Autodesk Inventor part; units mm, degrees
(part 2 of 3)
  line L1044 (421.44, -35) -> (424.615, -35) projected
  line L1045 (421.44, -45) -> (421.44, -35) projected
  line L1046 (424.615, -45) -> (421.44, -45) projected
  line L1047 (424.615, -45) -> (424.615, -55) projected
  line L1048 (421.44, -55) -> (424.615, -55) projected
  line L1049 (421.44, -65) -> (421.44, -55) projected
  line L1050 (424.615, -65) -> (421.44, -65) projected
  line L1051 (424.615, -65) -> (424.615, -75) projected
  line L1052 (421.44, -75) -> (424.615, -75) projected
  line L1053 (421.44, -75) -> (421.44, -86.825) projected
  line L1054 (421.44, -86.825) -> (426.44, -86.825) projected
  line L1055 (426.44, -86.825) -> (426.44, -90) projected
  line L1056 (426.44, -90) -> (436.44, -90) projected
  line L1057 (436.44, -90) -> (436.44, -86.825) projected
  line L1058 (436.44, -86.825) -> (446.44, -86.825) projected
  line L1059 (446.44, -86.825) -> (446.44, -90) projected
  line L1060 (446.44, -90) -> (456.44, -90) projected
  line L1061 (456.44, -90) -> (456.44, -86.825) projected
  line L1062 (456.44, -86.825) -> (466.44, -86.825) projected
  line L1063 (466.44, -86.825) -> (466.44, -90) projected
  line L1064 (466.44, -90) -> (476.44, -90) projected
  line L1065 (476.44, -90) -> (476.44, -86.825) projected
  line L1066 (476.44, -86.825) -> (486.44, -86.825) projected
  line L1067 (486.44, -86.825) -> (486.44, -90) projected
  line L1068 (486.44, -90) -> (496.44, -90) projected
  line L1069 (496.44, -90) -> (496.44, -86.825) projected
  line L1070 (496.44, -86.825) -> (506.44, -86.825) projected
  line L1071 (506.44, -86.825) -> (506.44, -90) projected
  line L1072 (506.44, -90) -> (516.44, -90) projected
  line L1073 (516.44, -90) -> (516.44, -86.825) projected
  line L1074 (516.44, -86.825) -> (526.44, -86.825) projected
  line L1075 (526.44, -86.825) -> (526.44, -90) projected
  line L1076 (526.44, -90) -> (536.44, -90) projected
  line L1077 (536.44, -90) -> (536.44, -86.825) projected
  line L1078 (536.44, -86.825) -> (541.44, -86.825) projected
  line L1079 (541.44, -86.825) -> (541.44, -75) projected
  line L1080 (541.44, -75) -> (538.265, -75) projected
  line L1081 (538.265, -75) -> (538.265, -65) projected
  line L1082 (538.265, -65) -> (541.44, -65) projected
  line L1083 (541.44, -65) -> (541.44, -55) projected
  line L1084 (541.44, -55) -> (538.265, -55) projected
  line L1085 (538.265, -55) -> (538.265, -51.5) projected
  line L1086 (538.265, -51.5) -> (536.265, -51.5) projected
  line L1087 (536.265, -51.5) -> (536.265, -52.75) projected
  line L1088 (536.265, -52.75) -> (533.765, -52.75) projected
  line L1089 (533.765, -52.75) -> (533.765, -51.5) projected
  line L1090 (533.765, -51.5) -> (527.44, -51.5) projected
  line L1091 (527.44, -51.5) -> (527.44, -48.5) projected
  line L1092 (527.44, -48.5) -> (533.765, -48.5) projected
  line L1093 (533.765, -48.5) -> (533.765, -47.25) projected
  line L1094 (533.765, -47.25) -> (536.265, -47.25) projected
  line L1095 (536.265, -47.25) -> (536.265, -48.5) projected
  circle A30 centre (504.4372, -27.4451) radius 3 projected
  circle A31 centre (458.4428, 54) radius 3 projected
  circle A32 centre (504.4372, 27.4451) radius 3 projected
  circle A33 centre (458.4428, -54) radius 3 projected
  circle A34 centre (466.44, 8.175) radius 11 projected
  line L1096 (541.56, 86.945) -> (541.56, 74.88)
  line L1097 (541.56, 74.88) -> (538.385, 74.88)
  line L1098 (538.385, 74.88) -> (538.385, 65.12)
  line L1099 (538.385, 65.12) -> (541.56, 65.12)
  line L1100 (541.56, 65.12) -> (541.56, 54.88)
  line L1101 (541.56, 54.88) -> (538.385, 54.88)
  line L1102 (538.385, 54.88) -> (538.385, 51.38)
  line L1103 (538.385, 51.38) -> (536.145, 51.38)
  line L1104 (536.145, 51.38) -> (536.145, 52.63)
  line L1105 (536.145, 52.63) -> (533.885, 52.63)
  line L1106 (533.885, 52.63) -> (533.885, 51.38)
  line L1107 (533.885, 51.38) -> (527.56, 51.38)
  line L1108 (527.56, 51.38) -> (527.56, 48.62)
  line L1109 (527.56, 48.62) -> (533.885, 48.62)
  line L1110 (533.885, 48.62) -> (533.885, 47.37)
  line L1111 (533.885, 47.37) -> (536.145, 47.37)
  line L1112 (536.145, 47.37) -> (536.145, 48.62)
  line L1113 (536.145, 48.62) -> (538.385, 48.62)
  line L1114 (538.385, 48.62) -> (538.385, 45.12)
  line L1115 (538.385, 45.12) -> (541.56, 45.12)
  line L1116 (541.56, 45.12) -> (541.56, 34.88)
  line L1117 (541.56, 34.88) -> (538.385, 34.88)
  line L1118 (538.385, 34.88) -> (538.385, 25.12)
  line L1119 (538.385, 25.12) -> (541.56, 25.12)
  line L1120 (541.56, 25.12) -> (541.56, 14.88)
  line L1121 (541.56, 14.88) -> (538.385, 14.88)
  line L1122 (538.385, 14.88) -> (538.385, 5.12)
  line L1123 (538.385, 5.12) -> (541.56, 5.12)
  line L1124 (541.56, 5.12) -> (541.56, -5.12)
  line L1125 (541.56, -5.12) -> (538.385, -5.12)
  line L1126 (538.385, -5.12) -> (538.385, -14.88)
  line L1127 (538.385, -14.88) -> (541.56, -14.88)
  line L1128 (541.56, -14.88) -> (541.56, -25.12)
  line L1129 (541.56, -25.12) -> (538.385, -25.12)
  line L1130 (538.385, -25.12) -> (538.385, -34.88)
  line L1131 (538.385, -34.88) -> (541.56, -34.88)
  line L1132 (541.56, -34.88) -> (541.56, -45.12)
  line L1133 (541.56, -45.12) -> (538.385, -45.12)
  line L1134 (538.385, -45.12) -> (538.385, -48.62)
  line L1135 (538.385, -48.62) -> (536.145, -48.62)
  line L1136 (536.145, -48.62) -> (536.145, -47.37)
  line L1137 (536.145, -47.37) -> (533.885, -47.37)
  line L1138 (533.885, -47.37) -> (533.885, -48.62)
  line L1139 (533.885, -48.62) -> (527.56, -48.62)
  line L1140 (527.56, -48.62) -> (527.56, -51.38)
  line L1141 (527.56, -51.38) -> (533.885, -51.38)
  line L1142 (533.885, -51.38) -> (533.885, -52.63)
  line L1143 (533.885, -52.63) -> (536.145, -52.63)
  line L1144 (536.145, -52.63) -> (536.145, -51.38)
  line L1145 (536.145, -51.38) -> (538.385, -51.38)
  line L1146 (538.385, -51.38) -> (538.385, -54.88)
  line L1147 (538.385, -54.88) -> (541.56, -54.88)
  line L1148 (541.56, -54.88) -> (541.56, -65.12)
  line L1149 (541.56, -65.12) -> (538.385, -65.12)
  line L1150 (538.385, -65.12) -> (538.385, -74.88)
  line L1151 (538.385, -74.88) -> (541.56, -74.88)
  line L1152 (541.56, -74.88) -> (541.56, -86.945)
  line L1153 (541.56, -86.945) -> (536.56, -86.945)
  line L1154 (536.56, -86.945) -> (536.56, -90.12)
  line L1155 (536.56, -90.12) -> (526.32, -90.12)
  line L1156 (526.32, -90.12) -> (526.32, -86.945)
  line L1157 (526.32, -86.945) -> (516.56, -86.945)
  line L1158 (516.56, -86.945) -> (516.56, -90.12)
  line L1159 (516.56, -90.12) -> (506.32, -90.12)
  line L1160 (506.32, -90.12) -> (506.32, -86.945)
  line L1161 (506.32, -86.945) -> (496.56, -86.945)
  line L1162 (496.56, -86.945) -> (496.56, -90.12)
  line L1163 (496.56, -90.12) -> (486.32, -90.12)
  line L1164 (486.32, -90.12) -> (486.32, -86.945)
  line L1165 (486.32, -86.945) -> (476.56, -86.945)
  line L1166 (476.56, -86.945) -> (476.56, -90.12)
  line L1167 (476.56, -90.12) -> (466.32, -90.12)
  line L1168 (466.32, -90.12) -> (466.32, -86.945)
  line L1169 (466.32, -86.945) -> (456.56, -86.945)
  line L1170 (456.56, -86.945) -> (456.56, -90.12)
  line L1171 (456.56, -90.12) -> (446.32, -90.12)
  line L1172 (446.32, -90.12) -> (446.32, -86.945)
  line L1173 (446.32, -86.945) -> (436.56, -86.945)
  line L1174 (436.56, -86.945) -> (436.56, -90.12)
  line L1175 (436.56, -90.12) -> (426.32, -90.12)
  line L1176 (426.32, -90.12) -> (426.32, -86.945)
  line L1177 (426.32, -86.945) -> (421.32, -86.945)
  line L1178 (421.32, -86.945) -> (421.32, -74.88)
  line L1179 (421.32, -74.88) -> (424.495, -74.88)
  line L1180 (424.495, -74.88) -> (424.495, -65.12)
  line L1181 (424.495, -65.12) -> (421.32, -65.12)
  line L1182 (421.32, -65.12) -> (421.32, -54.88)
  line L1183 (421.32, -54.88) -> (424.495, -54.88)
  line L1184 (424.495, -54.88) -> (424.495, -45.12)
  line L1185 (424.495, -45.12) -> (421.32, -45.12)
  line L1186 (421.32, -45.12) -> (421.32, -34.88)
  line L1187 (421.32, -34.88) -> (424.495, -34.88)
  line L1188 (424.495, -34.88) -> (424.495, -25.12)
  line L1189 (424.495, -25.12) -> (421.32, -25.12)
  line L1190 (421.32, -25.12) -> (421.32, -14.88)
  line L1191 (421.32, -14.88) -> (424.495, -14.88)
  line L1192 (424.495, -14.88) -> (424.495, -5.12)
  line L1193 (424.495, -5.12) -> (421.32, -5.12)
  line L1194 (421.32, -5.12) -> (421.32, 5.12)
  line L1195 (421.32, 5.12) -> (424.495, 5.12)
  line L1196 (424.495, 5.12) -> (424.495, 14.88)
  line L1197 (424.495, 14.88) -> (421.32, 14.88)
  line L1198 (421.32, 14.88) -> (421.32, 25.12)
  line L1199 (421.32, 25.12) -> (424.495, 25.12)
  line L1200 (424.495, 25.12) -> (424.495, 34.88)
  line L1201 (424.495, 34.88) -> (421.32, 34.88)
  line L1202 (421.32, 34.88) -> (421.32, 45.12)
  line L1203 (421.32, 45.12) -> (424.495, 45.12)
  line L1204 (424.495, 45.12) -> (424.495, 54.88)
  line L1205 (424.495, 54.88) -> (421.32, 54.88)
  line L1206 (421.32, 54.88) -> (421.32, 65.12)
  line L1207 (421.32, 65.12) -> (424.495, 65.12)
  line L1208 (424.495, 65.12) -> (424.495, 74.88)
  line L1209 (424.495, 74.88) -> (421.32, 74.88)
  line L1210 (421.32, 74.88) -> (421.32, 86.945)
  line L1211 (421.32, 86.945) -> (426.32, 86.945)
  line L1212 (426.32, 86.945) -> (426.32, 90.12)
  line L1213 (426.32, 90.12) -> (436.56, 90.12)
  line L1214 (436.56, 90.12) -> (436.56, 86.945)
  line L1215 (436.56, 86.945) -> (446.32, 86.945)
  line L1216 (446.32, 86.945) -> (446.32, 90.12)
  line L1217 (446.32, 90.12) -> (456.56, 90.12)
  line L1218 (456.56, 90.12) -> (456.56, 86.945)
  line L1219 (456.56, 86.945) -> (466.32, 86.945)
  line L1220 (466.32, 86.945) -> (466.32, 90.12)
  line L1221 (466.32, 90.12) -> (476.56, 90.12)
  line L1222 (476.56, 90.12) -> (476.56, 86.945)
  line L1223 (476.56, 86.945) -> (486.32, 86.945)
  line L1224 (486.32, 86.945) -> (486.32, 90.12)
  line L1225 (486.32, 90.12) -> (496.56, 90.12)
  line L1226 (496.56, 90.12) -> (496.56, 86.945)
  line L1227 (496.56, 86.945) -> (506.32, 86.945)
  line L1228 (506.32, 86.945) -> (506.32, 90.12)
  line L1229 (506.32, 90.12) -> (516.56, 90.12)
  line L1230 (516.56, 90.12) -> (516.56, 86.945)
  line L1231 (516.56, 86.945) -> (526.32, 86.945)
  line L1232 (526.32, 86.945) -> (526.32, 90.12)
  line L1233 (526.32, 90.12) -> (536.56, 90.12)
  line L1234 (536.56, 90.12) -> (536.56, 86.945)
  line L1235 (536.56, 86.945) -> (541.56, 86.945)
  circle A35 centre (527.16, 0) radius 0.958
  circle A36 centre (519.54, 0) radius 0.958
  line L1236 (525.135, -13.215) -> (521.565, -13.215)
  line L1237 (521.565, -13.215) -> (521.565, -2.025)
  line L1238 (521.565, -2.025) -> (525.135, -2.025)
  line L1239 (525.135, -2.025) -> (525.135, -13.215)
  circle A37 centre (527.16, -15.24) radius 0.958
  circle A38 centre (519.54, -15.24) radius 1.198
  circle A39 centre (504.4372, 27.4451) radius 2.88
  circle A40 centre (504.4372, -27.4451) radius 2.88
  circle A41 centre (533.716, -59.1479) radius 0.958
  circle A42 centre (498.716, -59.1479) radius 0.958
  circle A43 centre (458.4428, 54) radius 2.88
  circle A44 centre (466.44, 8.175) radius 10.88
  line L1240 (404.895, -13.335) -> (401.085, -13.335) projected
  line L1241 (401.085, -13.335) -> (401.085, -1.905) projected
  line L1242 (401.085, -1.905) -> (404.895, -1.905) projected
  line L1243 (404.895, -1.905) -> (404.895, -13.335) projected
  circle A45 centre (399.18, -15.24) radius 1.078 projected
  circle A46 centre (406.8, 0) radius 1.078 projected
  circle A47 centre (406.8, -15.24) radius 1.078 projected
  circle A48 centre (399.18, 0) radius 1.078 projected
  line L1244 (415.905, -48.5) -> (417.905, -48.5) projected
  line L1245 (417.905, -48.5) -> (417.905, -45) projected
  line L1246 (417.905, -45) -> (421.08, -45) projected
  line L1247 (421.08, -45) -> (421.08, -35) projected
  line L1248 (421.08, -35) -> (417.905, -35) projected
  line L1249 (417.905, -35) -> (417.905, -25) projected
  line L1250 (417.905, -25) -> (421.08, -25) projected
  line L1251 (421.08, -25) -> (421.08, -15) projected
  line L1252 (421.08, -15) -> (417.905, -15) projected
  line L1253 (417.905, -15) -> (417.905, -5) projected
  line L1254 (417.905, -5) -> (421.08, -5) projected
  line L1255 (421.08, -5) -> (421.08, 5) projected
  line L1256 (421.08, 5) -> (417.905, 5) projected
  line L1257 (417.905, 5) -> (417.905, 15) projected
  line L1258 (417.905, 15) -> (421.08, 15) projected
  line L1259 (421.08, 15) -> (421.08, 25) projected
  line L1260 (421.08, 25) -> (417.905, 25) projected
  line L1261 (417.905, 25) -> (417.905, 35) projected
  line L1262 (417.905, 35) -> (421.08, 35) projected
  line L1263 (421.08, 35) -> (421.08, 45) projected
  line L1264 (421.08, 45) -> (417.905, 45) projected
  line L1265 (417.905, 45) -> (417.905, 48.5) projected
  line L1266 (417.905, 48.5) -> (415.905, 48.5) projected
  line L1267 (415.905, 48.5) -> (415.905, 47.25) projected
  line L1268 (415.905, 47.25) -> (413.405, 47.25) projected
  line L1269 (413.405, 47.25) -> (413.405, 48.5) projected
  line L1270 (413.405, 48.5) -> (407.08, 48.5) projected
  line L1271 (407.08, 48.5) -> (407.08, 51.5) projected
  line L1272 (407.08, 51.5) -> (413.405, 51.5) projected
  line L1273 (413.405, 51.5) -> (413.405, 52.75) projected
  line L1274 (413.405, 52.75) -> (415.905, 52.75) projected
  line L1275 (415.905, 52.75) -> (415.905, 51.5) projected
  line L1276 (415.905, 51.5) -> (417.905, 51.5) projected
  line L1277 (417.905, 51.5) -> (417.905, 55) projected
  line L1278 (417.905, 55) -> (421.08, 55) projected
  line L1279 (421.08, 55) -> (421.08, 65) projected
  line L1280 (421.08, 65) -> (417.905, 65) projected
  line L1281 (417.905, 65) -> (417.905, 75) projected
  line L1282 (417.905, 75) -> (421.08, 75) projected
  line L1283 (421.08, 75) -> (421.08, 86.825) projected
  line L1284 (416.08, 86.825) -> (421.08, 86.825) projected
  line L1285 (416.08, 90) -> (416.08, 86.825) projected
  line L1286 (406.08, 90) -> (416.08, 90) projected
  line L1287 (406.08, 86.825) -> (406.08, 90) projected
  line L1288 (406.08, 86.825) -> (396.08, 86.825) projected
  line L1289 (396.08, 90) -> (396.08, 86.825) projected
  line L1290 (386.08, 90) -> (396.08, 90) projected
  line L1291 (386.08, 86.825) -> (386.08, 90) projected
  line L1292 (386.08, 86.825) -> (376.08, 86.825) projected
  line L1293 (376.08, 90) -> (376.08, 86.825) projected
  line L1294 (366.08, 90) -> (376.08, 90) projected
  line L1295 (366.08, 86.825) -> (366.08, 90) projected
  line L1296 (366.08, 86.825) -> (356.08, 86.825) projected
  line L1297 (356.08, 90) -> (356.08, 86.825) projected
  line L1298 (346.08, 90) -> (356.08, 90) projected
  line L1299 (346.08, 86.825) -> (346.08, 90) projected
  line L1300 (346.08, 86.825) -> (336.08, 86.825) projected
  line L1301 (336.08, 90) -> (336.08, 86.825) projected
  line L1302 (326.08, 90) -> (336.08, 90) projected
  line L1303 (326.08, 86.825) -> (326.08, 90) projected
  line L1304 (326.08, 86.825) -> (316.08, 86.825) projected
  line L1305 (316.08, 90) -> (316.08, 86.825) projected
  line L1306 (306.08, 90) -> (316.08, 90) projected
  line L1307 (306.08, 86.825) -> (306.08, 90) projected
  line L1308 (306.08, 86.825) -> (301.08, 86.825) projected
  line L1309 (301.08, 75) -> (301.08, 86.825) projected
  line L1310 (304.255, 75) -> (301.08, 75) projected
  line L1311 (304.255, 75) -> (304.255, 65) projected
  line L1312 (301.08, 65) -> (304.255, 65) projected
  line L1313 (301.08, 55) -> (301.08, 65) projected
  line L1314 (304.255, 55) -> (301.08, 55) projected
  line L1315 (304.255, 55) -> (304.255, 45) projected
  line L1316 (301.08, 45) -> (304.255, 45) projected
  line L1317 (301.08, 35) -> (301.08, 45) projected
  line L1318 (304.255, 35) -> (301.08, 35) projected
  line L1319 (304.255, 35) -> (304.255, 25) projected
  line L1320 (301.08, 25) -> (304.255, 25) projected
  line L1321 (301.08, 15) -> (301.08, 25) projected
  line L1322 (304.255, 15) -> (301.08, 15) projected
  line L1323 (304.255, 15) -> (304.255, 5) projected
  line L1324 (301.08, 5) -> (304.255, 5) projected
  line L1325 (301.08, -5) -> (301.08, 5) projected
  line L1326 (304.255, -5) -> (301.08, -5) projected
  line L1327 (304.255, -5) -> (304.255, -15) projected
  line L1328 (301.08, -15) -> (304.255, -15) projected
  line L1329 (301.08, -25) -> (301.08, -15) projected
  line L1330 (304.255, -25) -> (301.08, -25) projected
  line L1331 (304.255, -25) -> (304.255, -35) projected
  line L1332 (301.08, -35) -> (304.255, -35) projected
  line L1333 (301.08, -45) -> (301.08, -35) projected
  line L1334 (304.255, -45) -> (301.08, -45) projected
  line L1335 (304.255, -45) -> (304.255, -55) projected
  line L1336 (301.08, -55) -> (304.255, -55) projected
  line L1337 (301.08, -65) -> (301.08, -55) projected
  line L1338 (304.255, -65) -> (301.08, -65) projected
  line L1339 (304.255, -65) -> (304.255, -75) projected
  line L1340 (301.08, -75) -> (304.255, -75) projected
  line L1341 (301.08, -75) -> (301.08, -86.825) projected
  line L1342 (301.08, -86.825) -> (306.08, -86.825) projected
  line L1343 (306.08, -86.825) -> (306.08, -90) projected
  line L1344 (306.08, -90) -> (316.08, -90) projected
  line L1345 (316.08, -90) -> (316.08, -86.825) projected
  line L1346 (316.08, -86.825) -> (326.08, -86.825) projected
  line L1347 (326.08, -86.825) -> (326.08, -90) projected
  line L1348 (326.08, -90) -> (336.08, -90) projected
  line L1349 (336.08, -90) -> (336.08, -86.825) projected
  line L1350 (336.08, -86.825) -> (346.08, -86.825) projected
  line L1351 (346.08, -86.825) -> (346.08, -90) projected
  line L1352 (346.08, -90) -> (356.08, -90) projected
  line L1353 (356.08, -90) -> (356.08, -86.825) projected
  line L1354 (356.08, -86.825) -> (366.08, -86.825) projected
  line L1355 (366.08, -86.825) -> (366.08, -90) projected
  line L1356 (366.08, -90) -> (376.08, -90) projected
  line L1357 (376.08, -90) -> (376.08, -86.825) projected
  line L1358 (376.08, -86.825) -> (386.08, -86.825) projected
  line L1359 (386.08, -86.825) -> (386.08, -90) projected
  line L1360 (386.08, -90) -> (396.08, -90) projected
  line L1361 (396.08, -90) -> (396.08, -86.825) projected
  line L1362 (396.08, -86.825) -> (406.08, -86.825) projected
  line L1363 (406.08, -86.825) -> (406.08, -90) projected
  line L1364 (406.08, -90) -> (416.08, -90) projected
  line L1365 (416.08, -90) -> (416.08, -86.825) projected
  line L1366 (416.08, -86.825) -> (421.08, -86.825) projected
  line L1367 (421.08, -86.825) -> (421.08, -75) projected
  line L1368 (421.08, -75) -> (417.905, -75) projected
  line L1369 (417.905, -75) -> (417.905, -65) projected
  line L1370 (417.905, -65) -> (421.08, -65) projected
  line L1371 (421.08, -65) -> (421.08, -55) projected
  line L1372 (421.08, -55) -> (417.905, -55) projected
  line L1373 (417.905, -55) -> (417.905, -51.5) projected
  line L1374 (417.905, -51.5) -> (415.905, -51.5) projected
  line L1375 (415.905, -51.5) -> (415.905, -52.75) projected
  line L1376 (415.905, -52.75) -> (413.405, -52.75) projected
  line L1377 (413.405, -52.75) -> (413.405, -51.5) projected
  line L1378 (413.405, -51.5) -> (407.08, -51.5) projected
  line L1379 (407.08, -51.5) -> (407.08, -48.5) projected
  line L1380 (407.08, -48.5) -> (413.405, -48.5) projected
  line L1381 (413.405, -48.5) -> (413.405, -47.25) projected
  line L1382 (413.405, -47.25) -> (415.905, -47.25) projected
  line L1383 (415.905, -47.25) -> (415.905, -48.5) projected
  circle A49 centre (384.0772, -27.4451) radius 3 projected
  circle A50 centre (338.0828, 54) radius 3 projected
  circle A51 centre (384.0772, 27.4451) radius 3 projected
  circle A52 centre (338.0828, -54) radius 3 projected
  circle A53 centre (346.08, 8.175) radius 11 projected
  line L1384 (284.4, 59.88) -> (197.04, 59.88)
  line L1385 (197.04, 59.88) -> (197.04, -59.88)
  line L1386 (197.04, -59.88) -> (284.4, -59.88)
  line L1387 (284.4, -59.88) -> (284.4, 59.88)
  line L1388 (265.6, 90.12) -> (275.84, 90.12)
  line L1389 (275.84, 90.12) -> (275.84, 86.945)
  line L1390 (275.84, 86.945) -> (285.6, 86.945)
  line L1391 (285.6, 86.945) -> (285.6, 90.12)
  line L1392 (285.6, 90.12) -> (295.84, 90.12)
  line L1393 (295.84, 90.12) -> (295.84, 86.945)
  line L1394 (295.84, 86.945) -> (297.665, 86.945)
  line L1395 (297.665, 86.945) -> (297.665, 75.12)
  line L1396 (297.665, 75.12) -> (300.84, 75.12)
  line L1397 (300.84, 75.12) -> (300.84, 64.88)
  line L1398 (300.84, 64.88) -> (297.665, 64.88)
  line L1399 (297.665, 64.88) -> (297.665, 55.12)
  line L1400 (297.665, 55.12) -> (300.84, 55.12)
  line L1401 (300.84, 55.12) -> (300.84, 44.88)
  line L1402 (300.84, 44.88) -> (297.665, 44.88)
  line L1403 (297.665, 44.88) -> (297.665, 35.12)
  line L1404 (297.665, 35.12) -> (300.84, 35.12)
  line L1405 (300.84, 35.12) -> (300.84, 24.88)
  line L1406 (300.84, 24.88) -> (297.665, 24.88)
  line L1407 (297.665, 24.88) -> (297.665, 15.12)
  line L1408 (297.665, 15.12) -> (300.84, 15.12)
  line L1409 (300.84, 15.12) -> (300.84, 4.88)
  line L1410 (300.84, 4.88) -> (297.665, 4.88)
  line L1411 (297.665, 4.88) -> (297.665, -4.88)
  line L1412 (297.665, -4.88) -> (300.84, -4.88)
  line L1413 (300.84, -4.88) -> (300.84, -15.12)
  line L1414 (300.84, -15.12) -> (297.665, -15.12)
  line L1415 (297.665, -15.12) -> (297.665, -24.88)
  line L1416 (297.665, -24.88) -> (300.84, -24.88)
  line L1417 (300.84, -24.88) -> (300.84, -35.12)
  line L1418 (300.84, -35.12) -> (297.665, -35.12)
  line L1419 (297.665, -35.12) -> (297.665, -44.88)
  line L1420 (297.665, -44.88) -> (300.84, -44.88)
  line L1421 (300.84, -44.88) -> (300.84, -55.12)
  line L1422 (300.84, -55.12) -> (297.665, -55.12)
  line L1423 (297.665, -55.12) -> (297.665, -64.88)
  line L1424 (297.665, -64.88) -> (300.84, -64.88)
  line L1425 (300.84, -64.88) -> (300.84, -75.12)
  line L1426 (300.84, -75.12) -> (297.665, -75.12)
  line L1427 (297.665, -75.12) -> (297.665, -86.945)
  line L1428 (297.665, -86.945) -> (295.84, -86.945)
  line L1429 (295.84, -86.945) -> (295.84, -90.12)
  line L1430 (295.84, -90.12) -> (285.6, -90.12)
  line L1431 (285.6, -90.12) -> (285.6, -86.945)
  line L1432 (285.6, -86.945) -> (275.84, -86.945)
  line L1433 (275.84, -86.945) -> (275.84, -90.12)
  line L1434 (275.84, -90.12) -> (265.6, -90.12)
  line L1435 (265.6, -90.12) -> (265.6, -86.945)
  line L1436 (265.6, -86.945) -> (255.84, -86.945)
  line L1437 (255.84, -86.945) -> (255.84, -90.12)
  line L1438 (255.84, -90.12) -> (245.6, -90.12)
  line L1439 (245.6, -90.12) -> (245.6, -86.945)
  line L1440 (245.6, -86.945) -> (235.84, -86.945)
  line L1441 (235.84, -86.945) -> (235.84, -90.12)
  line L1442 (235.84, -90.12) -> (225.6, -90.12)
  line L1443 (225.6, -90.12) -> (225.6, -86.945)
  line L1444 (225.6, -86.945) -> (215.84, -86.945)
  line L1445 (215.84, -86.945) -> (215.84, -90.12)
  line L1446 (215.84, -90.12) -> (205.6, -90.12)
  line L1447 (205.6, -90.12) -> (205.6, -86.945)
  line L1448 (205.6, -86.945) -> (195.84, -86.945)
  line L1449 (195.84, -86.945) -> (195.84, -90.12)
  line L1450 (195.84, -90.12) -> (185.6, -90.12)
  line L1451 (185.6, -90.12) -> (185.6, -86.945)
  line L1452 (185.6, -86.945) -> (183.775, -86.945)
  line L1453 (183.775, -86.945) -> (183.775, -75.12)
  line L1454 (183.775, -75.12) -> (180.6, -75.12)
  line L1455 (180.6, -75.12) -> (180.6, -64.88)
  line L1456 (180.6, -64.88) -> (183.775, -64.88)
  line L1457 (183.775, -64.88) -> (183.775, -55.12)
  line L1458 (183.775, -55.12) -> (180.6, -55.12)
  line L1459 (180.6, -55.12) -> (180.6, -44.88)
  line L1460 (180.6, -44.88) -> (183.775, -44.88)
  line L1461 (183.775, -44.88) -> (183.775, -35.12)
  line L1462 (183.775, -35.12) -> (180.6, -35.12)
  line L1463 (180.6, -35.12) -> (180.6, -24.88)
  line L1464 (180.6, -24.88) -> (183.775, -24.88)
  line L1465 (183.775, -24.88) -> (183.775, -15.12)
  line L1466 (183.775, -15.12) -> (180.6, -15.12)
  line L1467 (180.6, -15.12) -> (180.6, -4.88)
  line L1468 (180.6, -4.88) -> (183.775, -4.88)
  line L1469 (183.775, -4.88) -> (183.775, 4.88)
  line L1470 (183.775, 4.88) -> (180.6, 4.88)
  line L1471 (180.6, 4.88) -> (180.6, 15.12)
  line L1472 (180.6, 15.12) -> (183.775, 15.12)
  line L1473 (183.775, 15.12) -> (183.775, 24.88)
  line L1474 (183.775, 24.88) -> (180.6, 24.88)
  line L1475 (180.6, 24.88) -> (180.6, 35.12)
  line L1476 (180.6, 35.12) -> (183.775, 35.12)
  line L1477 (183.775, 35.12) -> (183.775, 44.88)
  line L1478 (183.775, 44.88) -> (180.6, 44.88)
  line L1479 (180.6, 44.88) -> (180.6, 55.12)
  line L1480 (180.6, 55.12) -> (183.775, 55.12)
  line L1481 (183.775, 55.12) -> (183.775, 64.88)
  line L1482 (183.775, 64.88) -> (180.6, 64.88)
  line L1483 (180.6, 64.88) -> (180.6, 75.12)
  line L1484 (180.6, 75.12) -> (183.775, 75.12)
  line L1485 (183.775, 75.12) -> (183.775, 86.945)
  line L1486 (183.775, 86.945) -> (185.6, 86.945)
  line L1487 (185.6, 86.945) -> (185.6, 90.12)
  line L1488 (185.6, 90.12) -> (195.84, 90.12)
  line L1489 (195.84, 90.12) -> (195.84, 86.945)
  line L1490 (195.84, 86.945) -> (205.6, 86.945)
  line L1491 (205.6, 86.945) -> (205.6, 90.12)
  line L1492 (205.6, 90.12) -> (215.84, 90.12)
  line L1493 (215.84, 90.12) -> (215.84, 86.945)
  line L1494 (215.84, 86.945) -> (225.6, 86.945)
  line L1495 (225.6, 86.945) -> (225.6, 90.12)
  line L1496 (225.6, 90.12) -> (235.84, 90.12)
  line L1497 (235.84, 90.12) -> (235.84, 86.945)
  line L1498 (235.84, 86.945) -> (245.6, 86.945)
  line L1499 (245.6, 86.945) -> (245.6, 90.12)
  line L1500 (245.6, 90.12) -> (255.84, 90.12)
  line L1501 (255.84, 90.12) -> (255.84, 86.945)
  line L1502 (255.84, 86.945) -> (265.6, 86.945)
  line L1503 (265.6, 86.945) -> (265.6, 90.12)
  line L1504 (376.2, -90.48) -> (385.96, -90.48)
  line L1505 (385.96, -90.48) -> (385.96, -93.655)
  line L1506 (385.96, -93.655) -> (396.2, -93.655)
  line L1507 (396.2, -93.655) -> (396.2, -90.48)
  line L1508 (396.2, -90.48) -> (405.96, -90.48)
  line L1509 (405.96, -90.48) -> (405.96, -93.655)
  line L1510 (405.96, -93.655) -> (416.2, -93.655)
  line L1511 (416.2, -93.655) -> (416.2, -90.48)
  line L1512 (416.2, -90.48) -> (425.96, -90.48)
  line L1513 (425.96, -90.48) -> (425.96, -93.655)
  line L1514 (425.96, -93.655) -> (436.2, -93.655)
  line L1515 (436.2, -93.655) -> (436.2, -90.48)
  line L1516 (436.2, -90.48) -> (445.96, -90.48)
  line L1517 (445.96, -90.48) -> (445.96, -93.655)
  line L1518 (445.96, -93.655) -> (456.2, -93.655)
  line L1519 (456.2, -93.655) -> (456.2, -90.48)
  line L1520 (456.2, -90.48) -> (465.96, -90.48)
  line L1521 (465.96, -90.48) -> (465.96, -93.655)
  line L1522 (465.96, -93.655) -> (477.785, -93.655)
  line L1523 (477.785, -93.655) -> (477.785, -95.48)
  line L1524 (477.785, -95.48) -> (480.96, -95.48)
  line L1525 (480.96, -95.48) -> (480.96, -105.24)
  line L1526 (480.96, -105.24) -> (477.785, -105.24)
  line L1527 (477.785, -105.24) -> (477.785, -115.48)
  line L1528 (477.785, -115.48) -> (480.96, -115.48)
  line L1529 (480.96, -115.48) -> (480.96, -125.24)
  line L1530 (480.96, -125.24) -> (477.785, -125.24)
  line L1531 (477.785, -125.24) -> (477.785, -135.48)
  line L1532 (477.785, -135.48) -> (480.96, -135.48)
  line L1533 (480.96, -135.48) -> (480.96, -145.24)
  line L1534 (480.96, -145.24) -> (477.785, -145.24)
  line L1535 (477.785, -145.24) -> (477.785, -155.48)
  line L1536 (477.785, -155.48) -> (480.96, -155.48)
  line L1537 (480.96, -155.48) -> (480.96, -165.24)
  line L1538 (480.96, -165.24) -> (477.785, -165.24)
  line L1539 (477.785, -165.24) -> (477.785, -175.48)
  line L1540 (477.785, -175.48) -> (480.96, -175.48)
  line L1541 (480.96, -175.48) -> (480.96, -185.24)
  line L1542 (480.96, -185.24) -> (477.785, -185.24)
  line L1543 (477.785, -185.24) -> (477.785, -195.48)
  line L1544 (477.785, -195.48) -> (480.96, -195.48)
  line L1545 (480.96, -195.48) -> (480.96, -205.24)
  line L1546 (480.96, -205.24) -> (477.785, -205.24)
  line L1547 (477.785, -205.24) -> (477.785, -207.065)
  line L1548 (477.785, -207.065) -> (465.96, -207.065)
  line L1549 (465.96, -207.065) -> (465.96, -210.24)
  line L1550 (465.96, -210.24) -> (456.2, -210.24)
  line L1551 (456.2, -210.24) -> (456.2, -207.065)
  line L1552 (456.2, -207.065) -> (445.96, -207.065)
  line L1553 (445.96, -207.065) -> (445.96, -210.24)
  line L1554 (445.96, -210.24) -> (436.2, -210.24)
  line L1555 (436.2, -210.24) -> (436.2, -207.065)
  line L1556 (436.2, -207.065) -> (425.96, -207.065)
  line L1557 (425.96, -207.065) -> (425.96, -210.24)
  line L1558 (425.96, -210.24) -> (416.2, -210.24)
  line L1559 (416.2, -210.24) -> (416.2, -207.065)
  line L1560 (416.2, -207.065) -> (405.96, -207.065)
  line L1561 (405.96, -207.065) -> (405.96, -210.24)
  line L1562 (405.96, -210.24) -> (396.2, -210.24)
  line L1563 (396.2, -210.24) -> (396.2, -207.065)
  line L1564 (396.2, -207.065) -> (385.96, -207.065)
  line L1565 (385.96, -207.065) -> (385.96, -210.24)
  line L1566 (385.96, -210.24) -> (376.2, -210.24)
  line L1567 (376.2, -210.24) -> (376.2, -207.065)
  line L1568 (376.2, -207.065) -> (365.96, -207.065)
  line L1569 (365.96, -207.065) -> (365.96, -210.24)
  line L1570 (365.96, -210.24) -> (356.2, -210.24)
  line L1571 (356.2, -210.24) -> (356.2, -207.065)
  line L1572 (356.2, -207.065) -> (345.96, -207.065)
  line L1573 (345.96, -207.065) -> (345.96, -210.24)
  line L1574 (345.96, -210.24) -> (336.2, -210.24)
  line L1575 (336.2, -210.24) -> (336.2, -207.065)
  line L1576 (336.2, -207.065) -> (325.96, -207.065)
  line L1577 (325.96, -207.065) -> (325.96, -210.24)
  line L1578 (325.96, -210.24) -> (316.2, -210.24)
  line L1579 (316.2, -210.24) -> (316.2, -207.065)
  line L1580 (316.2, -207.065) -> (304.375, -207.065)
  line L1581 (304.375, -207.065) -> (304.375, -205.24)
  line L1582 (304.375, -205.24) -> (301.2, -205.24)
  line L1583 (301.2, -205.24) -> (301.2, -195.48)
  line L1584 (301.2, -195.48) -> (304.375, -195.48)
  line L1585 (304.375, -195.48) -> (304.375, -185.24)
  line L1586 (304.375, -185.24) -> (301.2, -185.24)
  line L1587 (301.2, -185.24) -> (301.2, -175.48)
  line L1588 (301.2, -175.48) -> (304.375, -175.48)
  line L1589 (304.375, -175.48) -> (304.375, -165.24)
  line L1590 (304.375, -165.24) -> (301.2, -165.24)
  line L1591 (301.2, -165.24) -> (301.2, -155.48)
  line L1592 (301.2, -155.48) -> (304.375, -155.48)
  line L1593 (304.375, -155.48) -> (304.375, -145.24)
  line L1594 (304.375, -145.24) -> (301.2, -145.24)
  line L1595 (301.2, -145.24) -> (301.2, -135.48)
  line L1596 (301.2, -135.48) -> (304.375, -135.48)
  line L1597 (304.375, -135.48) -> (304.375, -125.24)
  line L1598 (304.375, -125.24) -> (301.2, -125.24)
  line L1599 (301.2, -125.24) -> (301.2, -115.48)
  line L1600 (301.2, -115.48) -> (304.375, -115.48)
  line L1601 (304.375, -115.48) -> (304.375, -105.24)
  line L1602 (304.375, -105.24) -> (301.2, -105.24)
  line L1603 (301.2, -105.24) -> (301.2, -95.48)
  line L1604 (301.2, -95.48) -> (304.375, -95.48)
  line L1605 (304.375, -95.48) -> (304.375, -93.655)
  line L1606 (304.375, -93.655) -> (316.2, -93.655)
  line L1607 (316.2, -93.655) -> (316.2, -90.48)
  line L1608 (316.2, -90.48) -> (325.96, -90.48)
  line L1609 (325.96, -90.48) -> (325.96, -93.655)
  line L1610 (325.96, -93.655) -> (336.2, -93.655)
  line L1611 (336.2, -93.655) -> (336.2, -90.48)
  line L1612 (336.2, -90.48) -> (345.96, -90.48)
  line L1613 (345.96, -90.48) -> (345.96, -93.655)
  line L1614 (345.96, -93.655) -> (356.2, -93.655)
  line L1615 (356.2, -93.655) -> (356.2, -90.48)
  line L1616 (356.2, -90.48) -> (365.96, -90.48)
  line L1617 (365.96, -90.48) -> (365.96, -93.655)
  line L1618 (365.96, -93.655) -> (376.2, -93.655)
  line L1619 (376.2, -93.655) -> (376.2, -90.48)
  line L1620 (450.96, -106.68) -> (331.2, -106.68)
  line L1621 (331.2, -106.68) -> (331.2, -194.04)
  line L1622 (331.2, -194.04) -> (450.96, -194.04)
  line L1623 (450.96, -194.04) -> (450.96, -106.68)
  line L1624 (295.6, -207.305) -> (295.6, -210.48)
  line L1625 (295.6, -210.48) -> (300.84, -210.48)
  line L1626 (300.84, -210.48) -> (300.84, -205.24)
  line L1627 (300.84, -205.24) -> (297.665, -205.24)
  line L1628 (297.665, -205.24) -> (297.665, -195.48)
  line L1629 (297.665, -195.48) -> (300.84, -195.48)
  line L1630 (300.84, -195.48) -> (300.84, -185.24)
  line L1631 (300.84, -185.24) -> (297.665, -185.24)
  line L1632 (297.665, -185.24) -> (297.665, -175.48)
  line L1633 (297.665, -175.48) -> (300.84, -175.48)
  line L1634 (300.84, -175.48) -> (300.84, -165.24)
  line L1635 (300.84, -165.24) -> (297.665, -165.24)
  line L1636 (297.665, -165.24) -> (297.665, -155.48)
  line L1637 (297.665, -155.48) -> (300.84, -155.48)
  line L1638 (300.84, -155.48) -> (300.84, -145.24)
  line L1639 (300.84, -145.24) -> (297.665, -145.24)
  line L1640 (297.665, -145.24) -> (297.665, -135.48)
  line L1641 (297.665, -135.48) -> (300.84, -135.48)
  line L1642 (300.84, -135.48) -> (300.84, -125.24)
  line L1643 (300.84, -125.24) -> (297.665, -125.24)
  line L1644 (297.665, -125.24) -> (297.665, -115.48)
  line L1645 (297.665, -115.48) -> (300.84, -115.48)
  line L1646 (300.84, -115.48) -> (300.84, -105.24)
  line L1647 (300.84, -105.24) -> (297.665, -105.24)
  line L1648 (297.665, -105.24) -> (297.665, -95.48)
  line L1649 (297.665, -95.48) -> (300.84, -95.48)
  line L1650 (300.84, -95.48) -> (300.84, -90.24)
  line L1651 (300.84, -90.24) -> (295.6, -90.24)
  line L1652 (295.6, -90.24) -> (295.6, -93.415)
  line L1653 (295.6, -93.415) -> (285.84, -93.415)
  line L1654 (285.84, -93.415) -> (285.84, -90.24)
  line L1655 (285.84, -90.24) -> (275.6, -90.24)
  line L1656 (275.6, -90.24) -> (275.6, -93.415)
  line L1657 (275.6, -93.415) -> (265.84, -93.415)
  line L1658 (265.84, -93.415) -> (265.84, -90.24)
  line L1659 (265.84, -90.24) -> (255.6, -90.24)
  line L1660 (255.6, -90.24) -> (255.6, -93.415)
  line L1661 (255.6, -93.415) -> (245.84, -93.415)
  line L1662 (245.84, -93.415) -> (245.84, -90.24)
  line L1663 (245.84, -90.24) -> (235.6, -90.24)
  line L1664 (235.6, -90.24) -> (235.6, -93.415)
  line L1665 (235.6, -93.415) -> (225.84, -93.415)
  line L1666 (225.84, -93.415) -> (225.84, -90.24)
  line L1667 (225.84, -90.24) -> (215.6, -90.24)
  line L1668 (215.6, -90.24) -> (215.6, -93.415)
  line L1669 (215.6, -93.415) -> (205.84, -93.415)
  line L1670 (205.84, -93.415) -> (205.84, -90.24)
  line L1671 (205.84, -90.24) -> (195.6, -90.24)
  line L1672 (195.6, -90.24) -> (195.6, -93.415)
  line L1673 (195.6, -93.415) -> (185.84, -93.415)
  line L1674 (185.84, -93.415) -> (185.84, -90.24)
  line L1675 (185.84, -90.24) -> (180.6, -90.24)
  line L1676 (180.6, -90.24) -> (180.6, -95.48)
  line L1677 (180.6, -95.48) -> (183.775, -95.48)
  line L1678 (183.775, -95.48) -> (183.775, -105.24)
  line L1679 (183.775, -105.24) -> (180.6, -105.24)
  line L1680 (180.6, -105.24) -> (180.6, -115.48)
  line L1681 (180.6, -115.48) -> (183.775, -115.48)
  line L1682 (183.775, -115.48) -> (183.775, -125.24)
  line L1683 (183.775, -125.24) -> (180.6, -125.24)
  line L1684 (180.6, -125.24) -> (180.6, -135.48)
  line L1685 (180.6, -135.48) -> (183.775, -135.48)
  line L1686 (183.775, -135.48) -> (183.775, -145.24)
  line L1687 (183.775, -145.24) -> (180.6, -145.24)
  line L1688 (180.6, -145.24) -> (180.6, -155.48)
  line L1689 (180.6, -155.48) -> (183.775, -155.48)
  line L1690 (183.775, -155.48) -> (183.775, -165.24)
  line L1691 (183.775, -165.24) -> (180.6, -165.24)
  line L1692 (180.6, -165.24) -> (180.6, -175.48)
  line L1693 (180.6, -175.48) -> (183.775, -175.48)
  line L1694 (183.775, -175.48) -> (183.775, -185.24)
  line L1695 (183.775, -185.24) -> (180.6, -185.24)
  line L1696 (180.6, -185.24) -> (180.6, -195.48)
  line L1697 (180.6, -195.48) -> (183.775, -195.48)
  line L1698 (183.775, -195.48) -> (183.775, -205.24)
  line L1699 (183.775, -205.24) -> (180.6, -205.24)
  line L1700 (180.6, -205.24) -> (180.6, -210.48)
  line L1701 (180.6, -210.48) -> (185.84, -210.48)
  line L1702 (185.84, -210.48) -> (185.84, -207.305)
  line L1703 (185.84, -207.305) -> (195.6, -207.305)
  line L1704 (195.6, -207.305) -> (195.6, -210.48)
  line L1705 (195.6, -210.48) -> (205.84, -210.48)
  line L1706 (205.84, -210.48) -> (205.84, -207.305)
  line L1707 (205.84, -207.305) -> (215.6, -207.305)
  line L1708 (215.6, -207.305) -> (215.6, -210.48)
  line L1709 (215.6, -210.48) -> (225.84, -210.48)
  line L1710 (225.84, -210.48) -> (225.84, -207.305)
  line L1711 (225.84, -207.305) -> (235.6, -207.305)
  line L1712 (235.6, -207.305) -> (235.6, -210.48)
  line L1713 (235.6, -210.48) -> (245.84, -210.48)
  line L1714 (245.84, -210.48) -> (245.84, -207.305)
  line L1715 (245.84, -207.305) -> (255.6, -207.305)
  line L1716 (255.6, -207.305) -> (255.6, -210.48)
  line L1717 (255.6, -210.48) -> (265.84, -210.48)
  line L1718 (265.84, -210.48) -> (265.84, -207.305)
  line L1719 (265.84, -207.305) -> (275.6, -207.305)
  line L1720 (275.6, -207.305) -> (275.6, -210.48)
  line L1721 (275.6, -210.48) -> (285.84, -210.48)
  line L1722 (285.84, -210.48) -> (285.84, -207.305)
  line L1723 (285.84, -207.305) -> (295.6, -207.305)
  line L1724 (145.48, -210.48) -> (135.24, -210.48)
  line L1725 (135.24, -210.48) -> (135.24, -207.305)
  line L1726 (135.24, -207.305) -> (125.48, -207.305)
  line L1727 (125.48, -207.305) -> (125.48, -210.48)
  line L1728 (125.48, -210.48) -> (115.24, -210.48)
  line L1729 (115.24, -210.48) -> (115.24, -207.305)
  line L1730 (115.24, -207.305) -> (105.48, -207.305)
  line L1731 (105.48, -207.305) -> (105.48, -210.48)
  line L1732 (105.48, -210.48) -> (95.24, -210.48)
  line L1733 (95.24, -210.48) -> (95.24, -207.305)
  line L1734 (95.24, -207.305) -> (85.48, -207.305)
  line L1735 (85.48, -207.305) -> (85.48, -210.48)
  line L1736 (85.48, -210.48) -> (75.24, -210.48)
  line L1737 (75.24, -210.48) -> (75.24, -207.305)
  line L1738 (75.24, -207.305) -> (65.48, -207.305)
  line L1739 (65.48, -207.305) -> (65.48, -210.48)
  line L1740 (65.48, -210.48) -> (60.24, -210.48)
  line L1741 (60.24, -210.48) -> (60.24, -205.24)
  line L1742 (60.24, -205.24) -> (63.415, -205.24)
  line L1743 (63.415, -205.24) -> (63.415, -195.48)
  line L1744 (63.415, -195.48) -> (60.24, -195.48)
  line L1745 (60.24, -195.48) -> (60.24, -185.24)
  line L1746 (60.24, -185.24) -> (63.415, -185.24)
  line L1747 (63.415, -185.24) -> (63.415, -175.48)
  line L1748 (63.415, -175.48) -> (60.24, -175.48)
  line L1749 (60.24, -175.48) -> (60.24, -165.24)
  line L1750 (60.24, -165.24) -> (63.415, -165.24)
  line L1751 (63.415, -165.24) -> (63.415, -155.48)
  line L1752 (63.415, -155.48) -> (60.24, -155.48)
  line L1753 (60.24, -155.48) -> (60.24, -145.24)
  line L1754 (60.24, -145.24) -> (63.415, -145.24)
  line L1755 (63.415, -145.24) -> (63.415, -135.48)
  line L1756 (63.415, -135.48) -> (60.24, -135.48)
  line L1757 (60.24, -135.48) -> (60.24, -125.24)
  line L1758 (60.24, -125.24) -> (63.415, -125.24)
  line L1759 (63.415, -125.24) -> (63.415, -115.48)
  line L1760 (63.415, -115.48) -> (60.24, -115.48)
  line L1761 (60.24, -115.48) -> (60.24, -105.24)
  line L1762 (60.24, -105.24) -> (63.415, -105.24)
  line L1763 (63.415, -105.24) -> (63.415, -95.48)
  line L1764 (63.415, -95.48) -> (60.24, -95.48)
  line L1765 (60.24, -95.48) -> (60.24, -90.24)
  line L1766 (60.24, -90.24) -> (65.48, -90.24)
  line L1767 (65.48, -90.24) -> (65.48, -93.415)
  line L1768 (65.48, -93.415) -> (75.24, -93.415)
  line L1769 (75.24, -93.415) -> (75.24, -90.24)
  line L1770 (75.24, -90.24) -> (85.48, -90.24)
  line L1771 (85.48, -90.24) -> (85.48, -93.415)
  line L1772 (85.48, -93.415) -> (95.24, -93.415)
  line L1773 (95.24, -93.415) -> (95.24, -90.24)
  line L1774 (95.24, -90.24) -> (105.48, -90.24)
  line L1775 (105.48, -90.24) -> (105.48, -93.415)
  line L1776 (105.48, -93.415) -> (115.24, -93.415)
  line L1777 (115.24, -93.415) -> (115.24, -90.24)
  line L1778 (115.24, -90.24) -> (125.48, -90.24)
  line L1779 (125.48, -90.24) -> (125.48, -93.415)
  line L1780 (125.48, -93.415) -> (135.24, -93.415)
  line L1781 (135.24, -93.415) -> (135.24, -90.24)
  line L1782 (135.24, -90.24) -> (145.48, -90.24)
  line L1783 (145.48, -90.24) -> (145.48, -93.415)
  line L1784 (145.48, -93.415) -> (155.24, -93.415)
  line L1785 (155.24, -93.415) -> (155.24, -90.24)
  line L1786 (155.24, -90.24) -> (165.48, -90.24)
  line L1787 (165.48, -90.24) -> (165.48, -93.415)
  line L1788 (165.48, -93.415) -> (175.24, -93.415)
  line L1789 (175.24, -93.415) -> (175.24, -90.24)
  line L1790 (175.24, -90.24) -> (180.48, -90.24)
  line L1791 (180.48, -90.24) -> (180.48, -95.48)
  line L1792 (180.48, -95.48) -> (177.305, -95.48)
  line L1793 (177.305, -95.48) -> (177.305, -105.24)
  line L1794 (177.305, -105.24) -> (180.48, -105.24)
  line L1795 (180.48, -105.24) -> (180.48, -115.48)
  line L1796 (180.48, -115.48) -> (177.305, -115.48)
  line L1797 (177.305, -115.48) -> (177.305, -125.24)
  line L1798 (177.305, -125.24) -> (180.48, -125.24)
  line L1799 (180.48, -125.24) -> (180.48, -135.48)
  line L1800 (180.48, -135.48) -> (177.305, -135.48)
  line L1801 (177.305, -135.48) -> (177.305, -145.24)
  line L1802 (177.305, -145.24) -> (180.48, -145.24)
  line L1803 (180.48, -145.24) -> (180.48, -155.48)
  line L1804 (180.48, -155.48) -> (177.305, -155.48)
  line L1805 (177.305, -155.48) -> (177.305, -165.24)
  line L1806 (177.305, -165.24) -> (180.48, -165.24)
  line L1807 (180.48, -165.24) -> (180.48, -175.48)
  line L1808 (180.48, -175.48) -> (177.305, -175.48)
  line L1809 (177.305, -175.48) -> (177.305, -185.24)
  line L1810 (177.305, -185.24) -> (180.48, -185.24)
  line L1811 (180.48, -185.24) -> (180.48, -195.48)
  line L1812 (180.48, -195.48) -> (177.305, -195.48)
  line L1813 (177.305, -195.48) -> (177.305, -205.24)
  line L1814 (177.305, -205.24) -> (180.48, -205.24)
  line L1815 (180.48, -205.24) -> (180.48, -210.48)
  line L1816 (180.48, -210.48) -> (175.24, -210.48)
  line L1817 (175.24, -210.48) -> (175.24, -207.305)
  line L1818 (175.24, -207.305) -> (165.48, -207.305)
  line L1819 (165.48, -207.305) -> (165.48, -210.48)
  line L1820 (165.48, -210.48) -> (155.24, -210.48)
  line L1821 (155.24, -210.48) -> (155.24, -207.305)
  line L1822 (155.24, -207.305) -> (145.48, -207.305)
  line L1823 (145.48, -207.305) -> (145.48, -210.48)
  line L1824 (5.12, -210.48) -> (-5.12, -210.48)
  line L1825 (-5.12, -210.48) -> (-5.12, -207.305)
  line L1826 (-5.12, -207.305) -> (-14.88, -207.305)
  line L1827 (-14.88, -207.305) -> (-14.88, -210.48)
  line L1828 (-14.88, -210.48) -> (-25.12, -210.48)
  line L1829 (-25.12, -210.48) -> (-25.12, -207.305)
  line L1830 (-25.12, -207.305) -> (-34.88, -207.305)
  line L1831 (-34.88, -207.305) -> (-34.88, -210.48)
  line L1832 (-34.88, -210.48) -> (-45.12, -210.48)
  line L1833 (-45.12, -210.48) -> (-45.12, -207.305)
  line L1834 (-45.12, -207.305) -> (-54.88, -207.305)
  line L1835 (-54.88, -207.305) -> (-54.88, -210.48)
  line L1836 (-54.88, -210.48) -> (-60.12, -210.48)
  line L1837 (-60.12, -210.48) -> (-60.12, -205.24)
  line L1838 (-60.12, -205.24) -> (-56.945, -205.24)
  line L1839 (-56.945, -205.24) -> (-56.945, -195.48)
  line L1840 (-56.945, -195.48) -> (-60.12, -195.48)
  line L1841 (-60.12, -195.48) -> (-60.12, -185.24)
  line L1842 (-60.12, -185.24) -> (-56.945, -185.24)
  line L1843 (-56.945, -185.24) -> (-56.945, -175.48)
  line L1844 (-56.945, -175.48) -> (-60.12, -175.48)
  line L1845 (-60.12, -175.48) -> (-60.12, -165.24)
  line L1846 (-60.12, -165.24) -> (-56.945, -165.24)
  line L1847 (-56.945, -165.24) -> (-56.945, -155.48)
  line L1848 (-56.945, -155.48) -> (-60.12, -155.48)
  line L1849 (-60.12, -155.48) -> (-60.12, -145.24)
  line L1850 (-60.12, -145.24) -> (-56.945, -145.24)
  line L1851 (-56.945, -145.24) -> (-56.945, -135.48)
  line L1852 (-56.945, -135.48) -> (-60.12, -135.48)
  line L1853 (-60.12, -135.48) -> (-60.12, -125.24)
  line L1854 (-60.12, -125.24) -> (-56.945, -125.24)
  line L1855 (-56.945, -125.24) -> (-56.945, -115.48)
  line L1856 (-56.945, -115.48) -> (-60.12, -115.48)
  line L1857 (-60.12, -115.48) -> (-60.12, -105.24)
  line L1858 (-60.12, -105.24) -> (-56.945, -105.24)
  line L1859 (-56.945, -105.24) -> (-56.945, -95.48)
  line L1860 (-56.945, -95.48) -> (-60.12, -95.48)
  line L1861 (-60.12, -95.48) -> (-60.12, -90.24)
  line L1862 (-60.12, -90.24) -> (-54.88, -90.24)
  line L1863 (-54.88, -90.24) -> (-54.88, -93.415)
  line L1864 (-54.88, -93.415) -> (-45.12, -93.415)
  line L1865 (-45.12, -93.415) -> (-45.12, -90.24)
  line L1866 (-45.12, -90.24) -> (-34.88, -90.24)
  line L1867 (-34.88, -90.24) -> (-34.88, -93.415)
  line L1868 (-34.88, -93.415) -> (-25.12, -93.415)
  line L1869 (-25.12, -93.415) -> (-25.12, -90.24)
  line L1870 (-25.12, -90.24) -> (-14.88, -90.24)
  line L1871 (-14.88, -90.24) -> (-14.88, -93.415)
  line L1872 (-14.88, -93.415) -> (-5.12, -93.415)
  line L1873 (-5.12, -93.415) -> (-5.12, -90.24)
  line L1874 (-5.12, -90.24) -> (5.12, -90.24)
  line L1875 (5.12, -90.24) -> (5.12, -93.415)
  line L1876 (5.12, -93.415) -> (14.88, -93.415)
  line L1877 (14.88, -93.415) -> (14.88, -90.24)
  line L1878 (14.88, -90.24) -> (25.12, -90.24)
  line L1879 (25.12, -90.24) -> (25.12, -93.415)
  line L1880 (25.12, -93.415) -> (34.88, -93.415)
  line L1881 (34.88, -93.415) -> (34.88, -90.24)
  line L1882 (34.88, -90.24) -> (45.12, -90.24)
  line L1883 (45.12, -90.24) -> (45.12, -93.415)
  line L1884 (45.12, -93.415) -> (54.88, -93.415)
  line L1885 (54.88, -93.415) -> (54.88, -90.24)
  line L1886 (54.88, -90.24) -> (60.12, -90.24)
  line L1887 (60.12, -90.24) -> (60.12, -95.48)
  line L1888 (60.12, -95.48) -> (56.945, -95.48)
  line L1889 (56.945, -95.48) -> (56.945, -105.24)
  line L1890 (56.945, -105.24) -> (60.12, -105.24)
  line L1891 (60.12, -105.24) -> (60.12, -115.48)
  line L1892 (60.12, -115.48) -> (56.945, -115.48)
  line L1893 (56.945, -115.48) -> (56.945, -125.24)
  line L1894 (56.945, -125.24) -> (60.12, -125.24)
  line L1895 (60.12, -125.24) -> (60.12, -135.48)
  line L1896 (60.12, -135.48) -> (56.945, -135.48)
  line L1897 (56.945, -135.48) -> (56.945, -145.24)
  line L1898 (56.945, -145.24) -> (60.12, -145.24)
  line L1899 (60.12, -145.24) -> (60.12, -155.48)
  line L1900 (60.12, -155.48) -> (56.945, -155.48)
  line L1901 (56.945, -155.48) -> (56.945, -165.24)
  line L1902 (56.945, -165.24) -> (60.12, -165.24)
  line L1903 (60.12, -165.24) -> (60.12, -175.48)
  line L1904 (60.12, -175.48) -> (56.945, -175.48)
  line L1905 (56.945, -175.48) -> (56.945, -185.24)
  line L1906 (56.945, -185.24) -> (60.12, -185.24)
  line L1907 (60.12, -185.24) -> (60.12, -195.48)
  line L1908 (60.12, -195.48) -> (56.945, -195.48)
  line L1909 (56.945, -195.48) -> (56.945, -205.24)
  line L1910 (56.945, -205.24) -> (60.12, -205.24)
  line L1911 (60.12, -205.24) -> (60.12, -210.48)
  line L1912 (60.12, -210.48) -> (54.88, -210.48)
  line L1913 (54.88, -210.48) -> (54.88, -207.305)
  line L1914 (54.88, -207.305) -> (45.12, -207.305)
  line L1915 (45.12, -207.305) -> (45.12, -210.48)
  line L1916 (45.12, -210.48) -> (34.88, -210.48)
  line L1917 (34.88, -210.48) -> (34.88, -207.305)
  line L1918 (34.88, -207.305) -> (25.12, -207.305)
  line L1919 (25.12, -207.305) -> (25.12, -210.48)
  line L1920 (25.12, -210.48) -> (14.88, -210.48)
  line L1921 (14.88, -210.48) -> (14.88, -207.305)
  line L1922 (14.88, -207.305) -> (5.12, -207.305)
  line L1923 (5.12, -207.305) -> (5.12, -210.48)
  line L1924 (-56.945, -14.88) -> (-56.945, -5.12)
  line L1925 (-56.945, -5.12) -> (-60.12, -5.12)
  line L1926 (-60.12, -5.12) -> (-60.12, 5.12)
  line L1927 (-60.12, 5.12) -> (-56.945, 5.12)
  line L1928 (-56.945, 5.12) -> (-56.945, 14.88)
  line L1929 (-56.945, 14.88) -> (-60.12, 14.88)
  line L1930 (-60.12, 14.88) -> (-60.12, 25.12)
  line L1931 (-60.12, 25.12) -> (-56.945, 25.12)
  line L1932 (-56.945, 25.12) -> (-56.945, 34.88)
  line L1933 (-56.945, 34.88) -> (-60.12, 34.88)
  line L1934 (-60.12, 34.88) -> (-60.12, 45.12)
  line L1935 (-60.12, 45.12) -> (-56.945, 45.12)
  line L1936 (-56.945, 45.12) -> (-56.945, 54.88)
  line L1937 (-56.945, 54.88) -> (-60.12, 54.88)
  line L1938 (-60.12, 54.88) -> (-60.12, 65.12)
  line L1939 (-60.12, 65.12) -> (-56.945, 65.12)
  line L1940 (-56.945, 65.12) -> (-56.945, 74.88)
  line L1941 (-56.945, 74.88) -> (-60.12, 74.88)
  line L1942 (-60.12, 74.88) -> (-60.12, 86.945)
  line L1943 (-60.12, 86.945) -> (-55.12, 86.945)
  line L1944 (-55.12, 86.945) -> (-55.12, 90.12)
  line L1945 (-55.12, 90.12) -> (-44.88, 90.12)
  line L1946 (-44.88, 90.12) -> (-44.88, 86.945)
  line L1947 (-44.88, 86.945) -> (-35.12, 86.945)
  line L1948 (-35.12, 86.945) -> (-35.12, 90.12)
  line L1949 (-35.12, 90.12) -> (-24.88, 90.12)
  line L1950 (-24.88, 90.12) -> (-24.88, 86.945)
  line L1951 (-24.88, 86.945) -> (-15.12, 86.945)
  line L1952 (-15.12, 86.945) -> (-15.12, 90.12)
  line L1953 (-15.12, 90.12) -> (-4.88, 90.12)
  line L1954 (-4.88, 90.12) -> (-4.88, 86.945)
  line L1955 (-4.88, 86.945) -> (4.88, 86.945)
  line L1956 (4.88, 86.945) -> (4.88, 90.12)
  line L1957 (4.88, 90.12) -> (15.12, 90.12)
  line L1958 (15.12, 90.12) -> (15.12, 86.945)
  line L1959 (15.12, 86.945) -> (24.88, 86.945)
  line L1960 (24.88, 86.945) -> (24.88, 90.12)
  line L1961 (24.88, 90.12) -> (35.12, 90.12)
  line L1962 (35.12, 90.12) -> (35.12, 86.945)
  line L1963 (35.12, 86.945) -> (44.88, 86.945)
  line L1964 (44.88, 86.945) -> (44.88, 90.12)
  line L1965 (44.88, 90.12) -> (55.12, 90.12)
  line L1966 (55.12, 90.12) -> (55.12, 86.945)
  line L1967 (55.12, 86.945) -> (60.12, 86.945)
  line L1968 (60.12, 86.945) -> (60.12, 74.88)
  line L1969 (60.12, 74.88) -> (56.945, 74.88)
  line L1970 (56.945, 74.88) -> (56.945, 65.12)
  line L1971 (56.945, 65.12) -> (60.12, 65.12)
  line L1972 (60.12, 65.12) -> (60.12, 54.88)
  line L1973 (60.12, 54.88) -> (56.945, 54.88)
  line L1974 (56.945, 54.88) -> (56.945, 51.38)
  line L1975 (56.945, 51.38) -> (54.705, 51.38)
  line L1976 (54.705, 51.38) -> (54.705, 52.63)
  line L1977 (54.705, 52.63) -> (52.445, 52.63)
  line L1978 (52.445, 52.63) -> (52.445, 51.38)
  line L1979 (52.445, 51.38) -> (46.12, 51.38)
  line L1980 (46.12, 51.38) -> (46.12, 48.62)
  line L1981 (46.12, 48.62) -> (52.445, 48.62)
  line L1982 (52.445, 48.62) -> (52.445, 47.37)
  line L1983 (52.445, 47.37) -> (54.705, 47.37)
  line L1984 (54.705, 47.37) -> (54.705, 48.62)
  line L1985 (54.705, 48.62) -> (56.945, 48.62)
  line L1986 (56.945, 48.62) -> (56.945, 45.12)
  line L1987 (56.945, 45.12) -> (60.12, 45.12)
  line L1988 (60.12, 45.12) -> (60.12, 34.88)
  line L1989 (60.12, 34.88) -> (56.945, 34.88)
  line L1990 (56.945, 34.88) -> (56.945, 25.12)
  line L1991 (56.945, 25.12) -> (60.12, 25.12)
  line L1992 (60.12, 25.12) -> (60.12, 14.88)
  line L1993 (60.12, 14.88) -> (56.945, 14.88)
  line L1994 (56.945, 14.88) -> (56.945, 5.12)
  line L1995 (56.945, 5.12) -> (60.12, 5.12)
  line L1996 (60.12, 5.12) -> (60.12, -5.12)
  line L1997 (60.12, -5.12) -> (56.945, -5.12)
  line L1998 (56.945, -5.12) -> (56.945, -14.88)
  line L1999 (56.945, -14.88) -> (60.12, -14.88)
  line L2000 (60.12, -14.88) -> (60.12, -25.12)
  line L2001 (60.12, -25.12) -> (56.945, -25.12)
  line L2002 (56.945, -25.12) -> (56.945, -34.88)
  line L2003 (56.945, -34.88) -> (60.12, -34.88)
  line L2004 (60.12, -34.88) -> (60.12, -45.12)
  line L2005 (60.12, -45.12) -> (56.945, -45.12)
  line L2006 (56.945, -45.12) -> (56.945, -48.62)
  line L2007 (56.945, -48.62) -> (54.705, -48.62)
  line L2008 (54.705, -48.62) -> (54.705, -47.37)
  line L2009 (54.705, -47.37) -> (52.445, -47.37)
  line L2010 (52.445, -47.37) -> (52.445, -48.62)
  line L2011 (52.445, -48.62) -> (46.12, -48.62)
  line L2012 (46.12, -48.62) -> (46.12, -51.38)
  line L2013 (46.12, -51.38) -> (52.445, -51.38)
  line L2014 (52.445, -51.38) -> (52.445, -52.63)
  line L2015 (52.445, -52.63) -> (54.705, -52.63)
  line L2016 (54.705, -52.63) -> (54.705, -51.38)
  line L2017 (54.705, -51.38) -> (56.945, -51.38)
  line L2018 (56.945, -51.38) -> (56.945, -54.88)
  line L2019 (56.945, -54.88) -> (60.12, -54.88)
  line L2020 (60.12, -54.88) -> (60.12, -65.12)
  line L2021 (60.12, -65.12) -> (56.945, -65.12)
  line L2022 (56.945, -65.12) -> (56.945, -74.88)
  line L2023 (56.945, -74.88) -> (60.12, -74.88)
  line L2024 (60.12, -74.88) -> (60.12, -86.945)